Autodesk Fusion 360 part; units mm, degrees
note: some values were not read from the file. Chosen so that the rebuilt part matches the saved one: which face or edge a step refers to. Set by a fixed rule: which sketch regions a step uses.
(part 2 of 3)
sketch "BluetoothFacade" plane through (0, 0, 0) normal (0, 0, 1) x (1, 0, 0)
  circle A0 centre (-17.018, 6.656) radius 0.5
  circle A1 centre (-17.018, 11.656) radius 0.5
  circle A2 centre (-1.524, 11.656) radius 0.5
  line L0 (-3.6417, 15.5725) -> (-11.1417, 15.5725)
  line L1 (-11.1417, 15.5725) -> (-11.1417, 13.0725)
  line L2 (-11.1417, 13.0725) -> (-3.6417, 13.0725)
  line L3 (-3.6417, 13.0725) -> (-3.6417, 15.5725)
  line L4 (-3.6417, 12.3725) -> (-11.1417, 12.3725)
  line L5 (-11.1417, 12.3725) -> (-11.1417, 9.8725)
  line L6 (-11.1417, 9.8725) -> (-3.6417, 9.8725)
  line L7 (-3.6417, 9.8725) -> (-3.6417, 12.3725)
  circle A3 centre (-7.3917, 14.3225) radius 0.4
  line L8 (-11.1417, 11.1225) -> (-3.6417, 11.1225) construction
  line L9 (-7.3917, 9.8725) -> (-3.6417, 12.3725) construction
  line L10 (-7.3917, 9.8725) -> (-11.1417, 12.3725) construction
  circle A4 centre (-5.5167, 11.1225) radius 0.4
  circle A5 centre (-9.2667, 11.1225) radius 0.4
  circle A6 centre (-11.9078, 12.5832) radius 0.4
  line L11 (-1.524, 14.156) -> (-3.6417, 14.156) construction
  line L12 (-1.524, 11.656) -> (-3.6417, 11.656) construction
  line L13 (-19.3606, 6.656) -> (-17.018, 6.656) construction
  line L14 (-29.7609, -8.8954) -> (10.8139, -8.8954)
  line L15 (-15.4011, -2.8172) -> (-15.4011, 16.5279) construction
  line L16 (-15.4011, 16.5279) -> (-1.524, 16.656) construction
  circle A7 centre (-16.8606, -5.1163) radius 0.5
  line L17 (-16.8606, -5.1163) -> (-14.3606, -5.1163) construction
  line L18 (-21.8606, -5.1163) -> (-19.3606, -5.1163) construction
  line L19 (-19.3606, -5.1163) -> (-16.8606, -5.1163) construction
  circle A8 centre (-21.8606, -5.1163) radius 0.5
  circle A9 centre (-19.3606, -5.1163) radius 0.5
  circle A10 centre (-14.3606, -5.1163) radius 0.5
  line L20 (-19.3606, -5.1163) -> (-19.3606, 6.656) construction
  line L21 (-21.8606, -5.1163) -> (-21.9553, 11.656) construction
  line L22 (-17.018, 11.656) -> (-21.9553, 11.656) construction
  line L23 (-16.8606, -5.1163) -> (-15.4011, -2.8172) construction
  line L24 (-14.3606, -5.1163) -> (-13.3311, -5.1163) construction
  line L25 (-13.3311, -5.1163) -> (-13.3311, 6.6244) construction
  circle A11 centre (-12.4078, 12.5832) radius 0.4
  line L26 (-12.4078, 12.5832) -> (-12.4078, 6.6244) construction
  line L27 (-12.4078, 6.6244) -> (-13.3311, 6.6244) construction
  circle A12 centre (-1.524, 14.156) radius 0.4
  line L28 (-16.5229, -5.3307) -> (-15.0011, -2.9335)
  line L29 (-15.0011, -2.9335) -> (-15.0011, 16.1316)
  line L30 (-15.0011, 16.1316) -> (-1.5203, 16.256)
  line L31 (-17.1983, -4.902) -> (-15.8011, -2.701)
  line L32 (-15.8011, -2.701) -> (-15.8011, 16.9242)
  line L33 (-15.8011, 16.9242) -> (-1.5277, 17.056)
  line L34 (-14.3606, -5.5163) -> (-12.9311, -5.5163)
  line L35 (-12.9311, -5.5163) -> (-12.9311, 6.2244)
  line L36 (-12.0078, 6.2244) -> (-12.9311, 6.2244)
  line L37 (-12.0078, 12.5832) -> (-12.0078, 6.2244)
  line L38 (-14.3606, -4.7163) -> (-13.7311, -4.7163)
  line L39 (-13.7311, -4.7163) -> (-13.7311, 7.0244)
  line L40 (-12.8078, 7.0244) -> (-13.7311, 7.0244)
  line L41 (-12.8078, 12.5832) -> (-12.8078, 7.0244)
  line L42 (-18.9606, -5.1163) -> (-18.9606, 6.256)
  line L43 (-18.9606, 6.256) -> (-17.018, 6.256)
  line L44 (-19.7606, -5.1163) -> (-19.7606, 7.056)
  line L45 (-19.7606, 7.056) -> (-17.018, 7.056)
  line L46 (-21.4606, -5.1141) -> (-21.553, 11.256)
  line L47 (-17.018, 11.256) -> (-21.553, 11.256)
  line L48 (-22.2606, -5.1186) -> (-22.3576, 12.056)
  line L49 (-17.018, 12.056) -> (-22.3576, 12.056)
  circle A13 centre (-1.524, 16.656) radius 0.4
  circle A14 centre (-1.524, 14.156) radius 0.4
  line L50 (-14.3606, -5.5163) -> (-14.3606, -4.7163)
  line L51 (-16.5229, -5.3307) -> (-17.1983, -4.902)
  line L52 (-18.9606, -5.1163) -> (-19.7606, -5.1163)
  line L53 (-21.4606, -5.1141) -> (-22.2606, -5.1186)
  line L54 (-17.018, 6.256) -> (-17.018, 7.056)
  line L55 (-17.018, 11.256) -> (-17.018, 12.056)
  line L56 (-1.524, 12.156) -> (-3.6417, 12.156)
  line L57 (-1.524, 11.156) -> (-3.6417, 11.156)
  line L58 (-1.524, 14.556) -> (-3.6417, 14.556)
  line L59 (-1.524, 13.756) -> (-3.6417, 13.756)
  line L60 (-12.0078, 12.5832) -> (-12.0078, 13.609)
  line L61 (-11.1417, 11.1225) -> (-12.4078, 11.1225) construction
  line L62 (-12.4078, 12.5832) -> (-12.4078, 14.3225) construction
  line L63 (-12.4078, 14.3225) -> (-11.1417, 14.3225) construction
  line L64 (-7.7917, 14.3225) -> (-7.3917, 14.3225) construction
  line L65 (-11.1417, 11.5225) -> (-12.4078, 11.5225)
  line L66 (-11.1417, 10.7225) -> (-12.4078, 10.7225)
  line L67 (-12.0078, 12.5832) -> (-12.0078, 13.9225)
  line L68 (-12.0078, 13.9225) -> (-11.1417, 13.9225)
  line L69 (-12.8078, 12.5832) -> (-12.8078, 14.7225)
  line L70 (-12.8078, 14.7225) -> (-11.1417, 14.7225)
  line L71 (-21.8606, -5.1163) -> (-21.8606, -8.8954) construction
  line L72 (-19.3606, -5.1163) -> (-19.3606, -8.8954) construction
  line L73 (-16.8606, -5.1163) -> (-16.8606, -8.8954) construction
  line L74 (-14.3606, -5.1163) -> (-14.3606, -8.8954) construction
  line L75 (-20.8606, -8.8954) -> (-20.8606, -5.6163)
  arc A15 (-20.8606, -5.6163) -> (-22.8606, -5.6163) centre (-21.8606, -5.6163) ccw
  line L76 (-22.8606, -5.6163) -> (-22.8606, -8.8954)
  arc A16 (-22.8606, -8.8954) -> (-20.8606, -8.8954) centre (-21.8606, -8.8954) ccw
  line L77 (-21.8606, -8.8954) -> (-21.8606, -5.6163) construction
  line L78 (-18.3606, -8.8954) -> (-18.3606, -5.6163)
  arc A17 (-18.3606, -5.6163) -> (-20.3606, -5.6163) centre (-19.3606, -5.6163) ccw
  line L79 (-20.3606, -5.6163) -> (-20.3606, -8.8954)
  arc A18 (-20.3606, -8.8954) -> (-18.3606, -8.8954) centre (-19.3606, -8.8954) ccw
  line L80 (-19.3606, -8.8954) -> (-19.3606, -5.6163) construction
  line L81 (-15.8606, -8.8954) -> (-15.8606, -5.6163)
  arc A19 (-15.8606, -5.6163) -> (-17.8606, -5.6163) centre (-16.8606, -5.6163) ccw
  line L82 (-17.8606, -5.6163) -> (-17.8606, -8.8954)
  arc A20 (-17.8606, -8.8954) -> (-15.8606, -8.8954) centre (-16.8606, -8.8954) ccw
  line L83 (-16.8606, -8.8954) -> (-16.8606, -5.6163) construction
  line L84 (-13.3606, -8.8954) -> (-13.3606, -5.5163)
  arc A21 (-13.3606, -5.5163) -> (-15.3606, -5.5163) centre (-14.3606, -5.5163) ccw
  line L85 (-15.3606, -5.5163) -> (-15.3606, -8.8954)
  arc A22 (-15.3606, -8.8954) -> (-13.3606, -8.8954) centre (-14.3606, -8.8954) ccw
  line L86 (-14.3606, -8.8954) -> (-14.3606, -5.5163) construction
  line L87 (-23.9349, -3.5626) -> (-1.6062, -3.4365)
  line L88 (-21.3223, -3.5479) -> (-21.4152, 12.8951)
  line L89 (-17.9819, 12.8951) -> (-17.8891, -3.5285)
  line L90 (-17.9124, 0.5856) -> (11.9175, 0.754)
  circle A23 centre (-21.8606, -5.6163) radius 0.5
  circle A24 centre (-19.3606, -5.6163) radius 0.5
  circle A25 centre (-16.8606, -5.6163) radius 0.5
  circle A26 centre (-14.3606, -5.6163) radius 0.5
  circle A27 centre (-12.8078, 12.5832) radius 0.4
  point P0 (-17.018, 11.656)
  point P1 (-17.018, 6.656)
  point P2 (-1.524, 16.656)
  point P3 (-1.524, 14.156)
  point P4 (-17.018, 12.156)
  point P5 (-1.524, 11.656)
  point P6 (-2.024, 11.656)
  point P7 (-7.3917, 11.1225)
  point P8 (-9.2667, 11.1225)
  point P9 (-5.5167, 11.1225)
  point P10 (-21.8606, -5.1163)
  point P11 (-14.3606, -5.1163)
  point P12 (-16.8606, -5.1163)
  point P13 (-19.3606, -5.1163)
  point P14 (-1.524, 14.556)
  point P15 (-1.524, 13.756)
  dimension "d323" = 7.5
  dimension "d324" = 2.5
  dimension "d325" = 7.5
  dimension "d326" = 2.5
  dimension "d327" = 0.8
  dimension "d328" = 0.8
  dimension "d329" = 0.8
  dimension "d330" = 0.8
  dimension "d334" = 2.5
  dimension "d335" = 0.8
  dimension "d336" = 0.4
  dimension "d338" = 0.4
  dimension "d340" = 0.4
  dimension "d342" = 0.4
  dimension "d353" = 0.4
  dimension "d355" = 0.4
  dimension "d463" = 2
  dimension "d464" = 2
  dimension "d465" = 2
  dimension "d466" = 2
  constraint coincident P0 A1.centre
  constraint coincident A1 P4
  constraint coincident P5 A2.centre
  constraint coincident A2 P6
  constraint horizontal L0
  constraint vertical L1
  constraint horizontal L2
  constraint vertical L3
  constraint horizontal L4
  constraint vertical L5
  constraint horizontal L6
  constraint vertical L7
  constraint midpoint L5 L8.start
  constraint midpoint L7 L8.end
  constraint midpoint L8 P7
  constraint midpoint L6 L9.start
  constraint midpoint L10 P8
  constraint midpoint L9 P9
  constraint coincident P9 A4.centre
  constraint coincident P8 A5.centre
  constraint coincident P3 L11.start
  constraint coincident L3 L11.end
  constraint coincident L7 L12.end
  constraint perpendicular L7 L12
  constraint perpendicular L3 L11
  constraint coincident P1 A0.centre
  constraint coincident P2 L16.end
  constraint coincident P10 L18.start
  constraint coincident P12 A7.centre
  constraint coincident P13 L18.end
  constraint coincident P11 L17.end
  constraint equal L17 L19
  constraint equal L17 L18
  constraint equal A7 A10
  constraint equal A9 A10
  constraint equal A8 A10
  constraint perpendicular L13 L20
  constraint parallel L17 L24
  constraint coincident A11.centre L26.start
  constraint perpendicular L25 L27
  constraint perpendicular L26 L27
  constraint coincident L33.end A13
  constraint tangent L33 A13
  constraint coincident P14 A14
  constraint perpendicular L38 L50
  constraint perpendicular L28 L51
  constraint perpendicular L44 L52
  constraint perpendicular L48 L53
  constraint perpendicular L45 L54
  constraint perpendicular L49 L55
  constraint coincident A2 L56.start
  constraint coincident L7 L56.end
  constraint tangent A2 L56
  constraint perpendicular L7 L56
  constraint coincident A2 L57.start
  constraint coincident L7 L57.end
  constraint tangent A2 L57
  constraint perpendicular L7 L57
  constraint coincident P14 L58.start
  constraint coincident L3 L58.end
  constraint tangent A12 L58
  constraint perpendicular L3 L58
  constraint coincident P15 L59.start
  constraint coincident L3 L59.end
  constraint tangent A12 L59
  constraint perpendicular L3 L59
  constraint coincident A11 L37.start
  constraint coincident L37 L60.start
  constraint tangent A11 L60
  constraint perpendicular L59 L60
  constraint coincident L26 L61.end
  constraint perpendicular L26 L61
  constraint perpendicular L61 L62
  constraint coincident A3.centre L64.end
  constraint perpendicular L1 L63
  constraint coincident L1 L63.end
  constraint coincident A3 L64.start
  constraint collinear L63 L64
  constraint coincident L14 L71.end
  constraint coincident L14 L72.end
  constraint coincident L14 L73.end
  constraint coincident L14 L74.end
  constraint perpendicular L18 L71
  constraint perpendicular L19 L72
  constraint perpendicular L17 L74
  constraint perpendicular L17 L73
  constraint tangent L75 A15
  constraint tangent A15 L76
  constraint parallel L75 L76
  constraint tangent L76 A16
  constraint tangent L75 A16
  constraint coincident L71 A15.centre
  constraint coincident A8 A15.centre
  constraint perpendicular L14 L77
  constraint coincident L71.end A16.centre
  constraint tangent L78 A17
  constraint tangent A17 L79
  constraint parallel L78 L79
  constraint tangent L79 A18
  constraint tangent L78 A18
  constraint coincident A9 A17.centre
  constraint coincident L72 A17.centre
  constraint perpendicular L14 L80
  constraint coincident L72.end A18.centre
  constraint tangent L81 A19
  constraint tangent A19 L82
  constraint parallel L81 L82
  constraint tangent L82 A20
  constraint tangent L81 A20
  constraint coincident A7 A19.centre
  constraint coincident L73 A19.centre
  constraint perpendicular L14 L83
  constraint coincident L73.end A20.centre
  constraint tangent L84 A21
  constraint tangent A21 L85
  constraint parallel L84 L85
  constraint tangent L85 A22
  constraint tangent L84 A22
  constraint coincident L34.start L50.start
  constraint perpendicular L34 L86
  constraint coincident L74.end A22.centre
  constraint perpendicular L48 L87
  constraint coincident L87 L88.start
  constraint perpendicular L87 L88
  constraint coincident L87 L89.end
  constraint perpendicular L87 L89
  constraint coincident L89 L90.start
  constraint perpendicular L89 L90
  constraint concentric A15 A23
  constraint coincident P10 A23
  constraint concentric A17 A24
  constraint coincident P13 A24
  constraint tangent L19 A24
  constraint concentric A19 A25
  constraint coincident P12 A25
  constraint coincident A10 A26.centre
  constraint coincident L86 A26.centre
  constraint coincident P11 A26
  constraint tangent L17 A26
  constraint coincident L41.start L69.start
  constraint coincident A11.centre A27
  constraint tangent L26 A27
  measures "d323" distance of L0.start L0.end
  measures "d324" distance of L0.start L2.end
  measures "d325" distance of L4.end L4.start
  measures "d326" distance of L6.end L4.start
  measures "d327" diameter of A3
  measures "d328" diameter of A4
  measures "d329" diameter of A5
  measures "d330" diameter of A6
  measures "d334" distance of P12 P11
  measures "d335" diameter of A11
  measures "d463" diameter of A15
  measures "d464" diameter of A17
  measures "d465" diameter of A19
  measures "d466" diameter of A21
move_body "Move27" bodies 1 to x (1, 0, 0) y (0, 1, 0) z (0, 0, 1) at (0, 0, -9)
sketch "JointsPin9" plane through (0, 0, 0) normal (0, 0, 1) x (1, 0, 0)
  line L0 (36.0092, 39.4631) -> (36.0092, -0.5369) construction
  line L1 (41.6342, 39.8881) -> (30.3842, 39.8881)
  line L2 (30.3842, 39.8881) -> (30.3842, 39.0381)
  line L3 (30.3842, 39.0381) -> (41.6342, 39.0381)
  line L4 (41.6342, 39.0381) -> (41.6342, 39.8881)
  line L5 (41.6342, 39.8881) -> (30.3842, 39.0381) construction
  line L6 (30.3842, 39.8881) -> (41.6342, 39.0381) construction
  line L7 (30.3842, 34.0381) -> (41.6342, 34.0381)
  line L8 (41.6342, 34.0381) -> (41.6342, 34.8881)
  line L9 (30.3842, 34.8881) -> (30.3842, 34.0381)
  line L10 (41.6342, 34.8881) -> (30.3842, 34.8881)
  line L11 (30.3842, 29.0381) -> (41.6342, 29.0381)
  line L12 (41.6342, 29.0381) -> (41.6342, 29.8881)
  line L13 (30.3842, 29.8881) -> (30.3842, 29.0381)
  line L14 (41.6342, 29.8881) -> (30.3842, 29.8881)
  line L15 (30.3842, 24.0381) -> (41.6342, 24.0381)
  line L16 (41.6342, 24.0381) -> (41.6342, 24.8881)
  line L17 (30.3842, 24.8881) -> (30.3842, 24.0381)
  line L18 (41.6342, 24.8881) -> (30.3842, 24.8881)
  line L19 (30.3842, 19.0381) -> (41.6342, 19.0381)
  line L20 (41.6342, 19.0381) -> (41.6342, 19.8881)
  line L21 (30.3842, 19.8881) -> (30.3842, 19.0381)
  line L22 (41.6342, 19.8881) -> (30.3842, 19.8881)
  line L23 (30.3842, 14.0381) -> (41.6342, 14.0381)
  line L24 (41.6342, 14.0381) -> (41.6342, 14.8881)
  line L25 (30.3842, 14.8881) -> (30.3842, 14.0381)
  line L26 (41.6342, 14.8881) -> (30.3842, 14.8881)
  line L27 (30.3842, 9.0381) -> (41.6342, 9.0381)
  line L28 (41.6342, 9.0381) -> (41.6342, 9.8881)
  line L29 (30.3842, 9.8881) -> (30.3842, 9.0381)
  line L30 (41.6342, 9.8881) -> (30.3842, 9.8881)
  line L31 (30.3842, 4.0381) -> (41.6342, 4.0381)
  line L32 (41.6342, 4.0381) -> (41.6342, 4.8881)
  line L33 (30.3842, 4.8881) -> (30.3842, 4.0381)
  line L34 (41.6342, 4.8881) -> (30.3842, 4.8881)
  line L35 (30.3842, -0.9619) -> (41.6342, -0.9619)
  line L36 (41.6342, -0.9619) -> (41.6342, -0.1119)
  line L37 (30.3842, -0.1119) -> (30.3842, -0.9619)
  line L38 (41.6342, -0.1119) -> (30.3842, -0.1119)
  line L39 (30.3842, 19.4631) -> (36.0092, 19.4631) construction
  line L40 (36.0092, 19.4631) -> (33.3592, 19.4631) construction
  line L41 (36.0092, 41.4631) -> (33.3592, 41.4631)
  line L42 (33.3592, 41.4631) -> (33.3592, -2.5369)
  line L43 (33.3592, -2.5369) -> (36.0092, -2.5369)
  line L44 (36.0092, -2.5369) -> (36.0092, 41.4631)
  line L45 (36.0092, 41.4631) -> (33.3592, -2.5369) construction
  line L46 (33.3592, 41.4631) -> (36.0092, -2.5369) construction
  line L47 (36.0092, 27.0525) -> (33.3592, 27.0525)
  point P0 (36.0092, 39.4631)
  point P1 (34.6842, 19.4631)
  dimension "d213" = 40
  dimension "d214" = 11.25
  dimension "d215" = 0.85
  dimension "d218" = 40
  dimension "d219" = 0
  dimension "d220" = 2.65
  dimension "d221" = 44
  constraint vertical L0
  constraint horizontal L1
  constraint perpendicular L1 L2
  constraint parallel L1 L3
  constraint parallel L2 L4
  constraint coincident L5 P0
  constraint coincident L6 P0
  constraint coincident P0 L0.start
  constraint midpoint L21 L39.start
  constraint midpoint L0 L39.end
  constraint perpendicular L0 L40
  constraint horizontal L41
  constraint perpendicular L41 L42
  constraint parallel L41 L43
  constraint parallel L42 L44
  constraint coincident L45 P1
  constraint coincident L46 P1
  constraint midpoint L40 P1
  constraint coincident L0 L47.start
  constraint coincident L44 L47.start
  constraint coincident L42 L47.end
  constraint perpendicular L42 L47
  measures "d213" distance of P0 L0.end
  measures "d214" distance of L2.end L3.end
  measures "d215" distance of L1.end L2.end
  measures "d220" distance of L39.end L40.end
  measures "d221" distance of L41.end L42.end
extrude "Extrude18" add sketch "JointsPin9" along normal blind 3 separate body makes body 10
extrude "Extrude19" add sketch "JointsPin9" along normal blind 3 separate body contours L18 L42 L44 L47 | L15 L18 L42 L44 | L15 L16 L18 L44 | L15 L17 L18 L42 | L15 L22 L42 L44 | L19 L22 L42 L44 | L19 L20 L22 L44 | L19 L21 L22 L42 | L19 L26 L42 L44 | L23 L26 L42 L44 | L23 L24 L26 L44 | L23 L25 L26 L42 | L23 L30 L42 L44 | L27 L30 L42 L44 | L27 L28 L30 L44 | L27 L29 L30 L42 | L27 L34 L42 L44 | L31 L34 L42 L44 | L31 L32 L34 L44 | L31 L33 L34 L42 | L31 L38 L42 L44 | L35 L38 L42 L44 | L35 L36 L38 L44 | L35 L37 L38 L42 | L35 L42 L43 L44 makes body 11
move_body "Move10" bodies 10 to x (1, 0, 0) y (0, 1, 0) z (0, 0, 1) at (-25.5267, -0.3283, 0)
sketch "JointsPin6" plane through (0, 0, 3) normal (0, 0, 1) x (-1, 0, 0)
  line L0 (-36.0092, -27.0525) -> (-33.3592, -27.0525)
  line L1 (-33.3592, -27.0525) -> (-33.3592, -24.8881)
  line L2 (-33.3592, -24.8881) -> (-30.3842, -24.8881)
  line L3 (-30.3842, -24.8881) -> (-30.3842, -24.0381)
  line L4 (-30.3842, -24.0381) -> (-33.3592, -24.0381)
  line L5 (-33.3592, -24.0381) -> (-33.3592, -19.8881)
  line L6 (-33.3592, -19.8881) -> (-30.3842, -19.8881)
  line L7 (-30.3842, -19.8881) -> (-30.3842, -19.0381)
  line L8 (-30.3842, -19.0381) -> (-33.3592, -19.0381)
  line L9 (-33.3592, -19.0381) -> (-33.3592, -14.8881)
  line L10 (-33.3592, -14.8881) -> (-30.3842, -14.8881)
  line L11 (-30.3842, -14.8881) -> (-30.3842, -14.0381)
  line L12 (-30.3842, -14.0381) -> (-33.3592, -14.0381)
  line L13 (-33.3592, -14.0381) -> (-33.3592, -9.8881)
  line L14 (-33.3592, -9.8881) -> (-30.3842, -9.8881)
  line L15 (-30.3842, -9.8881) -> (-30.3842, -9.0381)
  line L16 (-30.3842, -9.0381) -> (-33.3592, -9.0381)
  line L17 (-33.3592, -9.0381) -> (-33.3592, -4.8881)
  line L18 (-33.3592, -4.8881) -> (-30.3842, -4.8881)
  line L19 (-30.3842, -4.8881) -> (-30.3842, -4.0381)
  line L20 (-30.3842, -4.0381) -> (-33.3592, -4.0381)
  line L21 (-33.3592, -4.0381) -> (-33.3592, 0.1119)
  line L22 (-33.3592, 0.1119) -> (-30.3842, 0.1119)
  line L23 (-30.3842, 0.1119) -> (-30.3842, 0.9619)
  line L24 (-30.3842, 0.9619) -> (-33.3592, 0.9619)
  line L25 (-33.3592, 0.9619) -> (-33.3592, 2.5369)
  line L26 (-33.3592, 2.5369) -> (-36.0092, 2.5369)
  line L27 (-36.0092, 2.5369) -> (-36.0092, 0.9619)
  line L28 (-36.0092, 0.9619) -> (-41.6342, 0.9619)
  line L29 (-41.6342, 0.9619) -> (-41.6342, 0.1119)
  line L30 (-41.6342, 0.1119) -> (-36.0092, 0.1119)
  line L31 (-36.0092, 0.1119) -> (-36.0092, -4.0381)
  line L32 (-36.0092, -4.0381) -> (-41.6342, -4.0381)
  line L33 (-41.6342, -4.0381) -> (-41.6342, -4.8881)
  line L34 (-41.6342, -4.8881) -> (-36.0092, -4.8881)
  line L35 (-36.0092, -4.8881) -> (-36.0092, -9.0381)
  line L36 (-36.0092, -9.0381) -> (-41.6342, -9.0381)
  line L37 (-41.6342, -9.0381) -> (-41.6342, -9.8881)
  line L38 (-41.6342, -9.8881) -> (-36.0092, -9.8881)
  line L39 (-36.0092, -9.8881) -> (-36.0092, -14.0381)
  line L40 (-36.0092, -14.0381) -> (-41.6342, -14.0381)
  line L41 (-41.6342, -14.0381) -> (-41.6342, -14.8881)
  line L42 (-41.6342, -14.8881) -> (-36.0092, -14.8881)
  line L43 (-36.0092, -14.8881) -> (-36.0092, -19.0381)
  line L44 (-36.0092, -19.0381) -> (-41.6342, -19.0381)
  line L45 (-41.6342, -19.0381) -> (-41.6342, -19.8881)
  line L46 (-41.6342, -19.8881) -> (-36.0092, -19.8881)
  line L47 (-36.0092, -19.8881) -> (-36.0092, -24.0381)
  line L48 (-36.0092, -24.0381) -> (-41.6342, -24.0381)
  line L49 (-41.6342, -24.0381) -> (-41.6342, -24.8881)
  line L50 (-41.6342, -24.8881) -> (-36.0092, -24.8881)
  line L51 (-36.0092, -24.8881) -> (-36.0092, -27.0525)
move_body "Move11" bodies 11 to x (-1, 0, 0) y (0, 1, 0) z (0, 0, -1) at (60.7683, 0, 6)
move_body "Move14" bodies 10 to x (1, 0, 0) y (0, 1, 0) z (0, 0, 1) at (0, -0.4, 0)
move_body "Move15" bodies 10 11 to x (1, 0, 0) y (0, 1, 0) z (0, 0, 1) at (0, 0, 9)
move_body "Move16" bodies 11 to x (1, 0, 0) y (0, 1, 0) z (0, 0, 1) at (-5, 0, 0)
move_body "Move17" bodies 10 to x (1, 0, 0) y (0, 1, 0) z (0, 0, 1) at (5, 0, 0)
move_body "Move18" bodies 10 to x (1, 0, 0) y (0, 1, 0) z (0, 0, 1) at (-2, 0, 0)
move_body "Move19" bodies 11 to x (1, 0, 0) y (0, 1, 0) z (0, 0, 1) at (1, 0, 0)
move_body "Move22" bodies 11 to x (1, 0, 0) y (0, 1, 0) z (0, 0, 1) at (1, 0, 0)
move_body "Move24" bodies 11 to x (1, 0, 0) y (0, 1, 0) z (0, 0, 1) at (-1.5, 0, 0)
sketch "Sketch14" plane through (0, 0, 0) normal (0, 0, 1) x (1, 0, 0)
  line L0 (2.4939, 24.156) -> (7.2229, 19.9038) construction
  line L1 (2, 0) -> (2, 43.18) construction
  line L2 (3.0148, 29.1179) -> (7.3096, 26.0825) construction
  line L3 (2.5669, 19.1001) -> (5.2599, 13.6706) construction
  line L4 (-1.524, 29.1179) -> (3.0148, 29.1179) construction
  line L5 (-1.524, 24.156) -> (2.4939, 24.156) construction
  line L6 (-1.524, 19.1001) -> (2.5669, 19.1001) construction
  line L7 (-1.524, 18.7001) -> (-1.524, 19.5001)
  line L8 (-17.0322, 21.6559) -> (-25.2181, 21.615) construction
  line L9 (-17.0302, 21.2559) -> (-17.0342, 22.0559)
  line L10 (-1.524, 23.756) -> (-1.524, 24.556)
  line L11 (-1.524, 28.7179) -> (-1.524, 29.5179)
  line L12 (-1.524, 33.7562) -> (-1.524, 34.5562)
  line L13 (-1.524, 38.7242) -> (-1.524, 39.5242)
  line L14 (-1.524, 36.656) -> (3.587, 38.7405) construction
  line L15 (-17.018, 31.7274) -> (-21.8788, 33.1161) construction
  line L16 (-21.8788, 33.1161) -> (-21.8788, 37.1874) construction
  circle A0 centre (-22.142, 24.1987) radius 0.4
  circle A1 centre (3.3671, 26.1953) radius 0.4
  line L17 (-17.018, 19.156) -> (-23.1737, 15.1489) construction
  line L18 (-1.524, 34.1562) -> (7.4703, 37.4164) construction
  line L19 (-1.524, 39.1242) -> (-1.524, 48.808) construction
  line L20 (-17.018, 39.156) -> (-17.018, 48.661) construction
  line L21 (-1.524, 31.656) -> (5.7926, 31.656) construction
  circle A2 centre (3.4, 20.8847) radius 0.4
  line L22 (-26.1444, 9.0108) -> (-26.1618, 44.721) construction
  line L23 (-25.1531, 14.1511) -> (-34.5845, 14.1465) construction
  line L24 (-34.5845, 14.1465) -> (-34.5874, 20.1465) construction
  line L25 (-34.5862, 17.6465) -> (-26.1486, 17.6506)
  arc A3 (-26.1486, 17.6506) -> (-26.151, 22.6506) centre (-26.1498, 20.1506) ccw
  line L26 (-26.151, 22.6506) -> (-34.5886, 22.6465)
  arc A4 (-34.5886, 22.6465) -> (-34.5862, 17.6465) centre (-34.5874, 20.1465) ccw
  line L27 (-34.5874, 20.1465) -> (-26.1498, 20.1506) construction
  line L28 (-34.5874, 20.1465) -> (-34.5908, 27.1465) construction
  line L29 (-34.5908, 27.1465) -> (-34.5942, 34.1465) construction
  line L30 (-34.5896, 24.6465) -> (-26.152, 24.6506)
  arc A5 (-26.152, 24.6506) -> (-26.1545, 29.6506) centre (-26.1532, 27.1506) ccw
  line L31 (-26.1545, 29.6506) -> (-34.592, 29.6465)
  arc A6 (-34.592, 29.6465) -> (-34.5896, 24.6465) centre (-34.5908, 27.1465) ccw
  line L32 (-34.5908, 27.1465) -> (-26.1532, 27.1506) construction
  line L33 (-34.593, 31.6465) -> (-26.1554, 31.6506)
  arc A7 (-26.1554, 31.6506) -> (-26.1579, 36.6506) centre (-26.1566, 34.1506) ccw
  line L34 (-26.1579, 36.6506) -> (-34.5955, 36.6465)
  arc A8 (-34.5955, 36.6465) -> (-34.593, 31.6465) centre (-34.5942, 34.1465) ccw
  line L35 (-34.5942, 34.1465) -> (-26.1566, 34.1506) construction
  line L36 (-34.5942, 34.1465) -> (-34.5977, 41.1465) construction
  line L37 (-34.5964, 38.6465) -> (-26.1588, 38.6506)
  arc A9 (-26.1588, 38.6506) -> (-26.1613, 43.6506) centre (-26.1601, 41.1506) ccw
  line L38 (-26.1613, 43.6506) -> (-34.5989, 43.6465)
  arc A10 (-34.5989, 43.6465) -> (-34.5964, 38.6465) centre (-34.5977, 41.1465) ccw
  line L39 (-34.5977, 41.1465) -> (-26.1601, 41.1506) construction
  line L40 (-21.8788, 37.1874) -> (-24.9334, 40.3913) construction
  line L41 (-17.018, 29.156) -> (-26.0361, 32.3783) construction
  line L42 (-17.018, 26.6496) -> (-25.2201, 26.6086) construction
  line L43 (7.5977, 8.186) -> (7.5795, 45.5927) construction
  line L44 (5.9588, 11.9298) -> (17.0919, 11.9352) construction
  line L45 (17.0919, 11.9352) -> (17.0922, 11.4005) construction
  line L46 (17.0922, 11.4005) -> (17.0888, 18.4005) construction
  line L47 (17.0888, 18.4005) -> (17.0853, 25.4005) construction
  line L48 (17.0853, 25.4005) -> (17.0853, 32.4005) construction
  line L49 (17.0853, 32.4005) -> (17.0853, 39.4005) construction
  line L50 (17.0853, 39.4005) -> (17.0855, 46.4005) construction
  line L51 (17.0855, 46.4005) -> (17.0855, 53.4005) construction
  line L52 (17.0875, 20.9005) -> (7.5915, 20.8959)
  arc A11 (7.5915, 20.8959) -> (7.594, 15.8959) centre (7.5928, 18.3959) ccw
  line L53 (7.594, 15.8959) -> (17.09, 15.9005)
  arc A12 (17.09, 15.9005) -> (17.0875, 20.9005) centre (17.0888, 18.4005) ccw
  line L54 (17.0888, 18.4005) -> (7.5928, 18.3959) construction
  line L55 (17.0841, 27.9005) -> (7.5881, 27.8959)
  arc A13 (7.5881, 27.8959) -> (7.5906, 22.8959) centre (7.5893, 25.3959) ccw
  line L56 (7.5906, 22.8959) -> (17.0866, 22.9005)
  arc A14 (17.0866, 22.9005) -> (17.0841, 27.9005) centre (17.0853, 25.4005) ccw
  line L57 (17.0853, 25.4005) -> (7.5893, 25.3959) construction
  line L58 (17.0841, 34.9005) -> (7.5847, 34.8959)
  arc A15 (7.5847, 34.8959) -> (7.5871, 29.8959) centre (7.5859, 32.3959) ccw
  line L59 (7.5871, 29.8959) -> (17.0866, 29.9005)
  arc A16 (17.0866, 29.9005) -> (17.0841, 34.9005) centre (17.0853, 32.4005) ccw
  line L60 (17.0853, 32.4005) -> (7.5859, 32.3959) construction
  line L61 (17.0841, 41.9005) -> (7.5813, 41.8959)
  arc A17 (7.5813, 41.8959) -> (7.5837, 36.8959) centre (7.5825, 39.3959) ccw
  line L62 (7.5837, 36.8959) -> (17.0866, 36.9005)
  arc A18 (17.0866, 36.9005) -> (17.0841, 41.9005) centre (17.0853, 39.4005) ccw
  line L63 (17.0853, 39.4005) -> (7.5825, 39.3959) construction
  line L64 (17.0855, 46.4005) -> (6.5795, 46.3954) construction
  line L65 (0.3436, 47.1461) -> (7.8682, 55.6021)
  arc A19 (7.8682, 55.6021) -> (4.133, 58.9259) centre (6.0006, 57.264) ccw
  line L66 (4.133, 58.9259) -> (-3.3916, 50.4699)
  arc A20 (-3.3916, 50.4699) -> (0.3436, 47.1461) centre (-1.524, 48.808) ccw
  line L67 (-1.524, 48.808) -> (6.0006, 57.264) construction
  line L68 (7.9664, 44.3154) -> (18.4724, 51.3205)
  arc A21 (18.4724, 51.3205) -> (15.6986, 55.4806) centre (17.0855, 53.4005) ccw
  line L69 (15.6986, 55.4806) -> (5.1926, 48.4754)
  arc A22 (5.1926, 48.4754) -> (7.9664, 44.3154) centre (6.5795, 46.3954) ccw
  line L70 (6.5795, 46.3954) -> (17.0855, 53.4005) construction
  line L71 (5.9588, 11.9298) -> (16.7833, 6.2799) construction
  line L72 (3.587, 38.7405) -> (3.587, 46.3133) construction
  line L73 (3.587, 46.3133) -> (5.735, 46.3133) construction
  line L74 (-26.9209, 15.9189) -> (-34.617, 8.2227)
  arc A23 (-34.617, 8.2227) -> (-31.0815, 4.6872) centre (-32.8493, 6.4549) ccw
  line L75 (-31.0815, 4.6872) -> (-23.3853, 12.3833)
  arc A24 (-23.3853, 12.3833) -> (-26.9209, 15.9189) centre (-25.1531, 14.1511) ccw
  line L76 (-25.1531, 14.1511) -> (-32.8493, 6.4549) construction
  line L77 (4.1911, 10.162) -> (15.2258, -0.8728)
  arc A25 (15.2258, -0.8728) -> (18.7614, 2.6628) centre (16.9936, 0.895) ccw
  line L78 (18.7614, 2.6628) -> (7.7266, 13.6975)
  arc A26 (7.7266, 13.6975) -> (4.1911, 10.162) centre (5.9588, 11.9298) ccw
  line L79 (5.9588, 11.9298) -> (16.9936, 0.895) construction
  line L80 (-34.5977, 41.1465) -> (-34.6011, 48.1465) construction
  line L81 (-34.5998, 45.6465) -> (-23.0363, 45.6521)
  arc A27 (-23.0363, 45.6521) -> (-23.0387, 50.6521) centre (-23.0375, 48.1521) ccw
  line L82 (-23.0387, 50.6521) -> (-34.6023, 50.6465)
  arc A28 (-34.6023, 50.6465) -> (-34.5998, 45.6465) centre (-34.6011, 48.1465) ccw
  line L83 (-34.6011, 48.1465) -> (-23.0375, 48.1521) construction
  line L84 (-17.018, 48.661) -> (-21.9778, 48.661) construction
  line L85 (-1.124, 39.1242) -> (-1.124, 48.808)
  line L86 (-1.924, 39.1242) -> (-1.924, 48.808)
  circle A29 centre (-17.018, 24.156) radius 0.4
  line L87 (-18.542, 24.1987) -> (-17.018, 24.156) construction
  line L88 (-0.2131, 21.6852) -> (-1.524, 21.656) construction
  line L89 (0.1162, 26.656) -> (-1.524, 26.656) construction
  line L90 (-1.524, 27.056) -> (-1.524, 26.256)
  line L91 (-1.5329, 22.0559) -> (-1.5151, 21.2561)
  line L92 (-17.0068, 24.5558) -> (-17.0292, 23.7561)
  line L93 (-17.418, 39.156) -> (-16.618, 39.156)
  line L94 (-17.1526, 28.7793) -> (-16.8834, 29.5327)
  line L95 (-17.2362, 19.4912) -> (-16.7998, 18.8207)
  line L96 (-1.524, 31.256) -> (-1.524, 32.056)
  line L97 (-1.3877, 33.7801) -> (-1.6603, 34.5322)
  line L98 (-1.3729, 36.2856) -> (-1.675, 37.0264)
  line L99 (-1.924, 39.1242) -> (-1.124, 39.1242)
  line L100 (-1.924, 48.808) -> (-1.124, 48.808)
  line L101 (-17.02, 27.0496) -> (-17.016, 26.2496)
  line L102 (7.3096, 26.0825) -> (7.5893, 25.3959) construction
  line L103 (5.7926, 31.656) -> (7.5859, 32.3959) construction
  line L104 (7.4703, 37.4164) -> (7.5825, 39.3959) construction
  line L105 (5.735, 46.3133) -> (6.5795, 46.3954) construction
  line L106 (-23.0375, 48.1521) -> (-21.9778, 48.661) construction
  line L107 (-26.1601, 41.1506) -> (-24.9334, 40.3913) construction
  line L108 (-26.0361, 32.3783) -> (-26.1566, 34.1506) construction
  line L109 (-25.2201, 26.6086) -> (-26.1532, 27.1506) construction
  line L110 (-26.1498, 20.1506) -> (-25.2181, 21.615) construction
  line L111 (-25.1531, 14.1511) -> (-23.1737, 15.1489) construction
  line L112 (5.2599, 13.6706) -> (5.9588, 11.9298) construction
  line L113 (7.2229, 19.9038) -> (7.5928, 18.3959) construction
  line L114 (-1.524, 18.7001) -> (2.3188, 18.7001)
  line L115 (2.3188, 18.7001) -> (4.8946, 13.507)
  line L116 (4.8946, 13.507) -> (5.5876, 11.7808)
  line L117 (-1.524, 19.5001) -> (2.815, 19.5001)
  line L118 (2.815, 19.5001) -> (5.6253, 13.8342)
  line L119 (5.6253, 13.8342) -> (6.33, 12.0788)
  line L120 (-1.524, 23.756) -> (2.3405, 23.756)
  line L121 (2.3405, 23.756) -> (6.8638, 19.6888)
  line L122 (6.8638, 19.6888) -> (7.2043, 18.3006)
  line L123 (-1.524, 24.556) -> (2.6473, 24.556)
  line L124 (2.6473, 24.556) -> (7.582, 20.1188)
  line L125 (7.582, 20.1188) -> (7.9812, 18.4912)
  line L126 (-1.524, 29.5179) -> (3.1419, 29.5179)
  line L127 (3.1419, 29.5179) -> (7.6359, 26.3417)
  line L128 (7.6359, 26.3417) -> (7.9598, 25.5468)
  line L129 (-1.524, 28.7179) -> (2.8877, 28.7179)
  line L130 (2.8877, 28.7179) -> (6.9833, 25.8233)
  line L131 (6.9833, 25.8233) -> (7.2189, 25.245)
  line L132 (-1.524, 32.056) -> (5.7133, 32.056)
  line L133 (5.7133, 32.056) -> (7.4334, 32.7657)
  line L134 (-1.524, 31.256) -> (5.8718, 31.256)
  line L135 (5.8718, 31.256) -> (7.7385, 32.0261)
  line L136 (-1.3877, 33.7801) -> (7.8547, 37.1302)
  line L137 (7.8547, 37.1302) -> (7.9819, 39.3733)
  line L138 (-1.6603, 34.5322) -> (7.0859, 37.7025)
  line L139 (7.0859, 37.7025) -> (7.1832, 39.4185)
  line L140 (-1.675, 37.0264) -> (3.187, 39.0093)
  line L141 (3.187, 39.0093) -> (3.187, 46.7133)
  line L142 (3.187, 46.7133) -> (5.7156, 46.7133)
  line L143 (5.7156, 46.7133) -> (6.5408, 46.7935)
  line L144 (-1.3729, 36.2856) -> (3.987, 38.4716)
  line L145 (3.987, 38.4716) -> (3.987, 45.9133)
  line L146 (3.987, 45.9133) -> (5.7544, 45.9133)
  line L147 (5.7544, 45.9133) -> (6.6182, 45.9973)
  line L148 (-17.418, 39.156) -> (-17.418, 48.261)
  line L149 (-17.418, 48.261) -> (-21.8868, 48.261)
  line L150 (-22.8644, 47.7916) -> (-21.8868, 48.261)
  line L151 (-16.618, 39.156) -> (-16.618, 49.061)
  line L152 (-16.618, 49.061) -> (-22.0689, 49.061)
  line L153 (-23.2107, 48.5127) -> (-22.0689, 49.061)
  line L154 (-16.9081, 32.112) -> (-21.4788, 33.4178)
  line L155 (-21.4788, 33.4178) -> (-21.4788, 37.3476)
  line L156 (-21.4788, 37.3476) -> (-24.6793, 40.7044)
  line L157 (-25.9495, 41.4907) -> (-24.6793, 40.7044)
  line L158 (-17.1279, 31.3428) -> (-22.2788, 32.8144)
  line L159 (-22.2788, 32.8144) -> (-22.2788, 37.0273)
  line L160 (-22.2788, 37.0273) -> (-25.1876, 40.0781)
  line L161 (-26.3706, 40.8105) -> (-25.1876, 40.0781)
  line L162 (-16.8834, 29.5327) -> (-25.6548, 32.6668)
  line L163 (-25.6548, 32.6668) -> (-25.7576, 34.1778)
  line L164 (-17.1526, 28.7793) -> (-26.4174, 32.0897)
  line L165 (-26.4174, 32.0897) -> (-26.5557, 34.1235)
  line L166 (-17.016, 26.2496) -> (-25.3269, 26.2081)
  line L167 (-25.3269, 26.2081) -> (-26.3541, 26.8047)
  line L168 (-17.02, 27.0496) -> (-25.1133, 27.0092)
  line L169 (-25.1133, 27.0092) -> (-25.9523, 27.4965)
  line L170 (-17.0342, 22.0559) -> (-25.4384, 22.0139)
  line L171 (-26.4873, 20.3654) -> (-25.4384, 22.0139)
  line L172 (-17.0302, 21.2559) -> (-24.9978, 21.2161)
  line L173 (-25.8123, 19.9359) -> (-24.9978, 21.2161)
  line L174 (-17.2362, 19.4912) -> (-23.3735, 15.4962)
  line L175 (-25.3332, 14.5083) -> (-23.3735, 15.4962)
  line L176 (-16.7998, 18.8207) -> (-22.974, 14.8017)
  line L177 (-24.973, 13.7939) -> (-22.974, 14.8017)
  line L178 (5.5876, 11.7808) -> (6.33, 12.0788)
  line L179 (7.2043, 18.3006) -> (7.9812, 18.4912)
  line L180 (7.2189, 25.245) -> (7.9598, 25.5468)
  line L181 (7.7385, 32.0261) -> (7.4334, 32.7657)
  line L182 (7.9819, 39.3733) -> (7.1832, 39.4185)
  line L183 (6.6182, 45.9973) -> (6.5408, 46.7935)
  line L184 (-22.8644, 47.7916) -> (-23.2107, 48.5127)
  line L185 (-26.3706, 40.8105) -> (-25.9495, 41.4907)
  line L186 (-26.5557, 34.1235) -> (-25.7576, 34.1778)
  line L187 (-26.3541, 26.8047) -> (-25.9523, 27.4965)
  line L188 (-25.8123, 19.9359) -> (-26.4873, 20.3654)
  line L189 (-24.973, 13.7939) -> (-25.3332, 14.5083)
  line L190 (-17.1279, 31.3428) -> (-16.9081, 32.112)
  line L191 (-0.2131, 21.6852) -> (3.4, 20.8847) construction
  line L192 (0.1162, 26.656) -> (3.3671, 26.1953) construction
  line L193 (-18.542, 24.1987) -> (-22.142, 24.1987) construction
  line L194 (-18.5364, 24.5987) -> (-17.0068, 24.5558)
  line L195 (-18.5364, 24.5987) -> (-22.142, 24.5987)
  line L196 (-18.5476, 23.7987) -> (-17.0292, 23.7561)
  line L197 (-18.5476, 23.7987) -> (-22.142, 23.7987)
  line L198 (0.1444, 27.056) -> (-1.524, 27.056)
  line L199 (0.1444, 27.056) -> (3.4232, 26.5913)
  line L200 (0.088, 26.256) -> (-1.524, 26.256)
  line L201 (0.088, 26.256) -> (3.311, 25.7992)
  line L202 (-0.1737, 22.0862) -> (-1.5329, 22.0559)
  line L203 (-0.1737, 22.0862) -> (3.4865, 21.2752)
  line L204 (-0.2525, 21.2843) -> (-1.5151, 21.2561)
  line L205 (-0.2525, 21.2843) -> (3.3135, 20.4942)
  circle A30 centre (-22.142, 24.1987) radius 1.1
  line L206 (-21.042, 0) -> (-21.042, 43.18)
  circle A31 centre (3.4, 20.8847) radius 0.9
  line L207 (2.5, 0) -> (2.5, 43.18)
  circle A32 centre (3.3671, 26.1953) radius 0.8671
  point P0 (-1.524, 31.656)
  point P1 (-1.524, 21.656)
  point P2 (-1.524, 24.156)
  point P3 (-1.524, 19.1001)
  point P4 (-1.524, 39.1242)
  point P5 (-1.524, 14.156)
  point P6 (-1.524, 29.1179)
  point P7 (-1.524, 34.1562)
  point P8 (-1.524, 26.656)
  point P9 (-17.018, 26.6496)
  point P10 (-17.018, 31.7274)
  point P11 (-1.524, 36.656)
  point P12 (-17.018, 29.156)
  point P13 (-17.018, 19.156)
  point P14 (-17.018, 39.156)
  dimension "d405" = 0.4
  dimension "d406" = 0.4
  dimension "d407" = 0.4
  dimension "d408" = -0.4
  dimension "d409" = -0.4
  dimension "d410" = -0.4
  dimension "d491" = -0.4
  dimension "d492" = 0.4
  dimension "d508" = 0.8
  dimension "d509" = 0.8
  dimension "d511" = 0.8
  dimension "d514" = 6
  dimension "d515" = 5
  dimension "d516" = 7
  dimension "d517" = 7
  dimension "d518" = 5
  dimension "d519" = 5
  dimension "d520" = 7
  dimension "d521" = 5
  dimension "d523" = 7
  dimension "d528" = 5
  dimension "d529" = 5
  dimension "d530" = 5
  dimension "d531" = 5
  dimension "d533" = 5
  dimension "d534" = 5
  dimension "d536" = 5
  dimension "d537" = 5
  dimension "d538" = 7
  dimension "d539" = 5
  dimension "d546" = 0.4
  dimension "d547" = 0.4
  dimension "d548" = 0.4
  dimension "d550" = 0.4
  dimension "d551" = 0.4
  dimension "d552" = 0.4
  dimension "d553" = 0.4
  dimension "d554" = 0.4
  dimension "d567" = 0.4
  dimension "d568" = 0.4
  dimension "d569" = 0.4
  dimension "d575" = 0.4
  dimension "d577" = 0.4
  constraint coincident P2 L5.start
  constraint coincident P3 L6.start
  constraint perpendicular L1 L6
  constraint coincident P6 L4.start
  constraint perpendicular L1 L4
  constraint perpendicular L7 L117
  constraint perpendicular L10 L123
  constraint perpendicular L4 L11
  constraint coincident P11 L14.start
  constraint coincident P10 L15.start
  constraint coincident P13 L17.start
  constraint coincident P7 L18.start
  constraint coincident P4 L19.start
  constraint parallel L13 L19
  constraint coincident P14 L20.start
  constraint vertical L20
  constraint coincident P0 L21.start
  constraint perpendicular L22 L23
  constraint coincident L23.end L24.start
  constraint perpendicular L23 L24
  constraint tangent L25 A3
  constraint tangent A3 L26
  constraint parallel L25 L26
  constraint tangent L26 A4
  constraint tangent L25 A4
  constraint coincident L22 A3.centre
  constraint perpendicular L22 L27
  constraint coincident L24.end A4.centre
  constraint perpendicular L26 L28
  constraint parallel L28 L29
  constraint tangent L30 A5
  constraint tangent A5 L31
  constraint parallel L30 L31
  constraint tangent L31 A6
  constraint tangent L30 A6
  constraint coincident L22 A5.centre
  constraint perpendicular L22 L32
  constraint coincident L28.end L29.start
  constraint tangent L33 A7
  constraint tangent A7 L34
  constraint parallel L33 L34
  constraint tangent L34 A8
  constraint tangent L33 A8
  constraint coincident L22 A7.centre
  constraint perpendicular L22 L35
  constraint coincident L29.end A8.centre
  constraint perpendicular L34 L36
  constraint tangent L37 A9
  constraint tangent A9 L38
  constraint parallel L37 L38
  constraint tangent L38 A10
  constraint tangent L37 A10
  constraint coincident L22 A9.centre
  constraint perpendicular L22 L39
  constraint coincident L36.end A10.centre
  constraint coincident P12 L41.start
  constraint coincident P9 L42.start
  constraint perpendicular L43 L44
  constraint coincident L44.end L45.start
  constraint perpendicular L44 L45
  constraint parallel L45 L46
  constraint parallel L46 L47
  constraint vertical L48
  constraint parallel L48 L49
  constraint parallel L49 L51
  constraint equal L46 L47
  constraint equal L46 L48
  constraint equal L46 L49
  constraint equal L46 L50
  constraint equal L46 L51
  constraint tangent L52 A11
  constraint tangent A11 L53
  constraint parallel L52 L53
  constraint tangent L53 A12
  constraint tangent L52 A12
  constraint coincident L43 A11.centre
  constraint perpendicular L43 L54
  constraint coincident L46.end L47.start
  constraint tangent L55 A13
  constraint tangent A13 L56
  constraint parallel L55 L56
  constraint tangent L56 A14
  constraint tangent L55 A14
  constraint coincident L43 A13.centre
  constraint perpendicular L43 L57
  constraint coincident L47.end L48.start
  constraint tangent L58 A15
  constraint tangent A15 L59
  constraint parallel L58 L59
  constraint tangent L59 A16
  constraint tangent L58 A16
  constraint coincident L43 A15.centre
  constraint perpendicular L43 L60
  constraint coincident L48.end L49.start
  constraint tangent L61 A17
  constraint tangent A17 L62
  constraint parallel L61 L62
  constraint tangent L62 A18
  constraint tangent L61 A18
  constraint coincident L43 A17.centre
  constraint perpendicular L43 L63
  constraint coincident L49.end L50.start
  constraint perpendicular L43 L64
  constraint coincident L50.end L51.start
  constraint tangent L65 A19
  constraint tangent A19 L66
  constraint parallel L65 L66
  constraint tangent L66 A20
  constraint tangent L65 A20
  constraint coincident L19.end A20.centre
  constraint tangent L68 A21
  constraint tangent A21 L69
  constraint parallel L68 L69
  constraint tangent L69 A22
  constraint tangent L68 A22
  constraint coincident L51.end A21.centre
  constraint coincident L64.end A22.centre
  constraint coincident L44.start L71.start
  constraint vertical L72
  constraint perpendicular L72 L73
  constraint tangent L74 A23
  constraint tangent A23 L75
  constraint parallel L74 L75
  constraint tangent L75 A24
  constraint tangent L74 A24
  constraint coincident L23.start A24.centre
  constraint tangent L77 A25
  constraint tangent A25 L78
  constraint parallel L77 L78
  constraint tangent L78 A26
  constraint tangent L77 A26
  constraint perpendicular L39 L80
  constraint tangent L81 A27
  constraint tangent A27 L82
  constraint parallel L81 L82
  constraint tangent L82 A28
  constraint tangent L81 A28
  constraint perpendicular L22 L83
  constraint coincident L80.end A28.centre
  constraint perpendicular L20 L84
  constraint coincident A29.centre L87.end
  constraint coincident P1 L88.end
  constraint coincident P8 L89.end
  constraint perpendicular L90 L200
  constraint perpendicular L91 L204
  constraint perpendicular L92 L196
  constraint perpendicular L93 L151
  constraint perpendicular L94 L162
  constraint perpendicular L95 L176
  constraint perpendicular L96 L132
  constraint perpendicular L97 L138
  constraint perpendicular L98 L140
  constraint perpendicular L85 L99
  constraint perpendicular L85 L100
  constraint perpendicular L101 L166
  constraint coincident A13.centre L57.end
  constraint coincident A15.centre L60.end
  constraint coincident A17.centre L63.end
  constraint coincident A27.centre L83.end
  constraint coincident A9.centre L39.end
  constraint coincident A7.centre L35.end
  constraint coincident A5.centre L32.end
  constraint coincident A3.centre L27.end
  constraint coincident A11.centre L54.end
  constraint perpendicular L119 L178
  constraint perpendicular L125 L179
  constraint perpendicular L131 L180
  constraint perpendicular L135 L181
  constraint perpendicular L139 L182
  constraint perpendicular L143 L183
  constraint perpendicular L153 L184
  constraint perpendicular L157 L185
  constraint perpendicular L163 L186
  constraint perpendicular L169 L187
  constraint perpendicular L171 L188
  constraint perpendicular L111 L189
  constraint perpendicular L154 L190
  constraint coincident A2.centre L191.end
  constraint coincident A1.centre L192.end
  constraint coincident A0.centre L193.end
  constraint horizontal L193
  constraint concentric A0 A30
  constraint tangent A30 L206
  constraint tangent A31 L207
  constraint concentric A1 A32
  constraint tangent L207 A32
  measures "d508" diameter of A0
  measures "d509" diameter of A1
  measures "d511" diameter of A2
  measures "d514" distance of L23.end L24.end
  measures "d515" diameter of A3
  measures "d516" distance of L24.end L28.end
  measures "d517" distance of L28.end L29.end
  measures "d518" diameter of A5
  measures "d519" diameter of A7
  measures "d520" distance of L29.end L36.end
  measures "d521" diameter of A9
  measures "d523" distance of L45.end L46.end
  measures "d528" diameter of A11
  measures "d529" diameter of A13
  measures "d530" diameter of A15
  measures "d531" diameter of A17
  measures "d533" diameter of A19
  measures "d534" diameter of A21
  measures "d536" diameter of A23
  measures "d537" diameter of A25
  measures "d538" distance of L36.end L80.end
  measures "d539" diameter of A27
move_body "Move29" bodies 1 to x (1, 0, 0) y (0, 1, 0) z (0, 0, 1) at (0, 0, 9)
extrude "Extrude41" cut sketch "BluetoothFacade" against normal blind 6 contours A0 L43 L45 L54 | A0 L43 L45 L54 | A0 L43 L45 L89 | L42 L43 L44 L45 L87 L89 | A1 L47 L49 L89 | L47 L49 L88 L89 | L42 L44 A17 L87 | A1 L47 L49 L55 | A1 L47 L49 L55 | L46 L47 L48 L49 L87 L88 | L28 L29 L31 L32 L87 L90 | L29 L30 L32 L33 A13 L90 | A9 L44 A17 | A9 L42 A17 | L28 L31 A19 L87 | A9 L44 L52 A24 | A9 L42 L44 L52 | L46 L48 A15 L87 | A9 L42 L52 A24 | A7 L31 A19 | A13 | L35 L39 L87 L90 | A6 A11 L35 L36 L37 L39 L40 L41 L90 A27 | A9 A24 | A8 L46 A15 | A7 L31 L51 A25 | A7 L28 L31 L51 A25 | A7 L28 A19 | L34 L35 L38 L39 A21 L87 | A8 A23 | A8 L46 L48 L53 | A8 L46 L53 A23 | A8 L48 A15 | A7 L28 L51 A25 | A7 L28 A25 | A8 L48 L53 A23 | L28 L51 A25 | A10 L34 L38 A21 A26 | A11 L41 A27 | A10 L38 L50 A26 | A10 L38 L50 A26 | A11 L69 A27 | A11 A27 | L1 A6 A11 L60 L67 L68 L69 L70 A27 | A6 A11 A27 | L5 L37 L65 L66 | A10 L34 L50 A26 | A10 L34 A26 | A6 A11 L37 | A6 A11 | L4 L5 L6 L7 | A10 L34 L50 A26 | A6 A11 L60 L67 | L0 L1 L2 L3 | A6 L37 L60 L67 | A2 L7 L56 L57 | L3 A12 A14 L58 L59 | A2 | A12 A14 | A3 | A4 | A5 picked at (-19.3854, -5.2849) picked at (-21.8854, -5.4478) picked at (-13.9529, -5.453) bodies 1
extrude "Extrude43" cut sketch "BluetoothFacade" against normal blind 7 contours A3 | A4 | A5 bodies 1
extrude "Extrude44" cut sketch "BluetoothFacade" against normal blind 9 contours L41 L69 A27 | A11 L41 A27 | A11 L69 A27 | A11 A27 | A6 A11 A27 | A6 A11 L37 | A6 A11 | A6 A11 L60 L67 | A6 L37 L60 L67 bodies 1
extrude "Extrude45" cut sketch "BluetoothFacade" against normal blind 9 contours A9 L44 L52 A24 | A9 L42 L44 L52 | A9 L42 L52 A24 | A9 A24 | A9 A24 | A7 L31 L51 A25 | A7 L28 L31 L51 A25 | A8 A23 | A8 L46 L48 L53 | A8 L46 L53 A23 | A7 L28 L51 A25 | A7 A25 | A7 L28 A25 | A8 L48 L53 A23 | L28 L51 A25 | A8 A23 | A10 L38 L50 A26 | A10 L38 L50 A26 | A10 L34 L50 A26 | A10 L34 A26 | A10 L34 A26 | A10 L34 L50 A26 bodies 1
extrude "Extrude46" cut sketch "ArduinoNano" against normal blind 9 contours A1 | A2 | A3 | A6 L199 | A6 L199 | A11 | A16 L51 L57 | A16 L51 L57 | A16 L51 | A19 | A23 | A24 L86 | A24 L86 | A26 | L43 L53 A44 | L43 L53 A44 | L43 L53 A44 | L43 L53 A44 | A30 | A33 | A40 | A41 | A43 | A48 L61 | A48 L61 | A49 | A56 | A57 | A60 | A63 | A67 | L109 A117 L176 | L109 A117 L176 | L109 A117 L176 | L109 A117 L176 | A91 | A98 | A114 | A116 | A123 | A124 | A130 | A131 | A132 | A136 | A141 | A143 bodies 1
extrude "Extrude47" cut sketch "ResistancesHolesTunnels" against normal blind 2.1 contours L76 L82 L84 L85 bodies 1
extrude "Extrude48" cut sketch "BluetoothFacade" against normal blind 6 contours L14 A9 L42 L44 L78 A17 L79 A24 | L14 A7 L28 L31 L81 A19 L82 A25 | A9 A24 | L14 A8 L46 L48 L75 A15 L76 A23 | A7 A25 | L14 A10 L34 L38 L84 A21 L85 A26 | A8 A23 | A10 L34 A26 picked at (-19.4166, -5.7782) picked at (-21.9166, -5.7782) picked at (-14.4089, -5.9463) bodies 1
move_body "Move30" bodies 1 to x (1, 0, 0) y (0, 1, 0) z (0, 0, 1) at (0, 0, 9)
move_body "Move31" bodies 1 to x (1, 0, 0) y (0, 1, 0) z (0, 0, 1) at (0, 0, -9)
extrude "Extrude50" cut sketch "BluetoothFacade" against normal blind 5 contours L14 A9 L42 L44 L78 A17 L79 A24 | L14 A7 L28 L31 L81 A19 L82 A25 | A9 A24 | L14 A8 L46 L48 L75 A15 L76 A23 | A7 A25 | L14 A10 L34 L38 L84 A21 L85 A26 | A8 A23 | A10 L34 A26 picked at (-19.4166, -5.7782) picked at (-21.9166, -5.7782) picked at (-14.4089, -5.9463) bodies 1
extrude "Extrude52" cut sketch "ArduinoNano" against normal blind 2.1 contours L202 L203 L204 L205 L206 L207 bodies 1
extrude "Extrude53" cut sketch "ResistancesHolesTunnels" against normal blind 4.1 contours L76 L82 L84 L85 | L82 L86 L90 L91 bodies 1